Autodesk Fusion 360 part; units mm, degrees
(part 2 of 3)
  spline S66 degree 5 poles (-69.4959, 44.6139) (-69.3858, 44.4624) (-69.2873, 44.0709) (-69.5097, 43.2258) (-70.5375, 41.634) (-72.8973, 39.0758) (-76.0944, 36.2068) (-79.8229, 33.3082) (-83.7318, 30.658) (-87.4483, 28.5038) (-90.6105, 27.0501) (-92.8999, 26.443) (-94.0756, 26.7557) (-94.0097, 27.9705) (-92.7249, 29.9603) (-90.3651, 32.5184) (-87.1679, 35.3874) (-83.4395, 38.286) (-79.5306, 40.9363) (-75.814, 43.0904) (-72.6519, 44.5442) (-70.8204, 45.0298) (-69.9479, 44.9801) (-69.606, 44.7654) (-69.4959, 44.6139) knots 0 0 0 0 0 0 0.05 0.1 0.15 0.2 0.25 0.3 0.35 0.4 0.45 0.5 0.55 0.6 0.65 0.7 0.75 0.8 0.85 0.9 0.95 1 1 1 1 1 1
  line L144 (-69.9146, 45.1902) -> (-69.0772, 44.0376)
  line L145 (-69.9146, 45.1902) -> (-69.0772, 44.0376)
  line L146 (-85.3889, 40.9075) -> (-85.5128, 41.2013)
  spline S67 degree 5 poles (-77.8115, 47.5528) (-77.808, 47.4659) (-77.8969, 47.2932) (-78.3187, 47.042) (-79.4326, 46.738) (-81.582, 46.4414) (-84.2579, 46.2523) (-87.1892, 46.1863) (-90.0921, 46.2497) (-92.6973, 46.4372) (-94.7656, 46.7338) (-96.1037, 47.1154) (-96.5801, 47.5501) (-96.1432, 47.9989) (-94.8404, 48.4163) (-92.7994, 48.7562) (-90.2109, 48.9784) (-87.312, 49.054) (-84.3725, 48.973) (-81.678, 48.7483) (-79.5015, 48.4089) (-78.3613, 48.0774) (-77.9183, 47.815) (-77.8151, 47.6398) (-77.8115, 47.5528) knots 0 0 0 0 0 0 0.05 0.1 0.15 0.2 0.25 0.3 0.35 0.4 0.45 0.5 0.55 0.6 0.65 0.7 0.75 0.8 0.85 0.9 0.95 1 1 1 1 1 1
  line L147 (-77.825, 47.881) -> (-77.7981, 47.2246)
  line L148 (-53.2432, 64.6583) -> (-52.9372, 64.4734)
  line L149 (-105.9017, 18.1636) -> (-105.9017, 76.9421)
  spline S68 degree 5 poles (-85.4509, 54.0512) (-85.4681, 54.0103) (-85.5538, 53.9424) (-85.8347, 53.8848) (-86.4976, 53.9022) (-87.715, 54.0845) (-89.1941, 54.4186) (-90.7877, 54.882) (-92.3423, 55.4366) (-93.7126, 56.0256) (-94.7704, 56.5824) (-95.4139, 57.0408) (-95.5768, 57.3449) (-95.2387, 57.4591) (-94.4366, 57.3785) (-93.2522, 57.1222) (-91.8004, 56.726) (-90.2181, 56.2359) (-88.6538, 55.702) (-87.2569, 55.1719) (-86.1659, 54.6895) (-85.6291, 54.3726) (-85.4501, 54.1882) (-85.4336, 54.0922) (-85.4509, 54.0512) knots 0 0 0 0 0 0 0.05 0.1 0.15 0.2 0.25 0.3 0.35 0.4 0.45 0.5 0.55 0.6 0.65 0.7 0.75 0.8 0.85 0.9 0.95 1 1 1 1 1 1
  line L150 (-85.3814, 54.2159) -> (-85.5203, 53.8865)
  spline S69 degree 5 poles (-60.4508, 47.5528) (-60.4508, 47.7401) (-60.3005, 48.1148) (-59.6238, 48.6678) (-57.8567, 49.3514) (-54.4439, 50.034) (-50.171, 50.4758) (-45.4508, 50.6293) (-40.7307, 50.4758) (-36.4578, 50.034) (-33.045, 49.3514) (-30.8361, 48.4969) (-30.0687, 47.5528) (-30.8361, 46.6088) (-33.045, 45.7542) (-36.4578, 45.0717) (-40.7307, 44.6299) (-45.4508, 44.4764) (-50.171, 44.6299) (-54.4439, 45.0717) (-57.8567, 45.7542) (-59.6238, 46.4379) (-60.3005, 46.9909) (-60.4508, 47.3655) (-60.4508, 47.5528) knots 0 0 0 0 0 0 0.05 0.1 0.15 0.2 0.25 0.3 0.35 0.4 0.45 0.5 0.55 0.6 0.65 0.7 0.75 0.8 0.85 0.9 0.95 1 1 1 1 1 1
  line L151 (-60.4508, 46.8405) -> (-60.4508, 48.2651)
  line L152 (-65.2797, 26.5381) -> (-65.622, 26.5091)
  line L153 (-85.3814, 54.2159) -> (-85.5203, 53.8865)
  spline S70 degree 5 poles (-65.4508, 26.5236) (-65.4952, 26.5198) (-65.5861, 26.4593) (-65.7277, 26.2099) (-65.916, 25.5741) (-66.1189, 24.36) (-66.2582, 22.85) (-66.3099, 21.1912) (-66.2628, 19.5413) (-66.1261, 18.0561) (-65.9235, 16.878) (-65.6864, 16.1243) (-65.4475, 15.8754) (-65.2344, 16.1617) (-65.0631, 16.9495) (-64.9409, 18.1551) (-64.8691, 19.6583) (-64.8463, 21.3145) (-64.8707, 22.9673) (-64.9431, 24.4596) (-65.0647, 25.6463) (-65.2003, 26.2547) (-65.3203, 26.4819) (-65.4065, 26.5273) (-65.4508, 26.5236) knots 0 0 0 0 0 0 0.05 0.1 0.15 0.2 0.25 0.3 0.35 0.4 0.45 0.5 0.55 0.6 0.65 0.7 0.75 0.8 0.85 0.9 0.95 1 1 1 1 1 1
  line L154 (-65.2797, 26.5381) -> (-65.622, 26.5091)
  line L155 (-100.9017, 21.7963) -> (-100.9017, 73.3094)
  line L156 (-77.9412, 64.4537) -> (-77.6818, 64.678)
  line L157 (-77.9468, 30.6568) -> (-77.6763, 30.4228)
  spline S71 degree 5 poles (-77.8115, 30.5398) (-77.7779, 30.5107) (-77.7398, 30.4083) (-77.7719, 30.1233) (-77.9933, 29.4982) (-78.5428, 28.3967) (-79.3177, 27.0933) (-80.2509, 25.7209) (-81.2587, 24.4138) (-82.2423, 23.2926) (-83.0987, 22.4585) (-83.7335, 21.9882) (-84.0731, 21.9272) (-84.0772, 22.2841) (-83.7527, 23.0221) (-83.143, 24.0693) (-82.3175, 25.3276) (-81.3624, 26.681) (-80.3712, 28.0037) (-79.4355, 29.1684) (-78.6395, 30.057) (-78.1723, 30.4696) (-77.9416, 30.5828) (-77.8452, 30.5689) (-77.8115, 30.5398) knots 0 0 0 0 0 0 0.05 0.1 0.15 0.2 0.25 0.3 0.35 0.4 0.45 0.5 0.55 0.6 0.65 0.7 0.75 0.8 0.85 0.9 0.95 1 1 1 1 1 1
  line L158 (-77.9468, 30.6568) -> (-77.6763, 30.4228)
  spline S72 degree 5 poles (-69.4959, 50.4918) (-69.606, 50.3402) (-69.9479, 50.1255) (-70.8204, 50.0759) (-72.6519, 50.5615) (-75.814, 52.0152) (-79.5306, 54.1694) (-83.4395, 56.8197) (-87.1679, 59.7182) (-90.3651, 62.5872) (-92.7249, 65.1454) (-94.0097, 67.1351) (-94.0756, 68.3499) (-92.8999, 68.6626) (-90.6105, 68.0556) (-87.4483, 66.6018) (-83.7318, 64.4477) (-79.8229, 61.7974) (-76.0944, 58.8988) (-72.8973, 56.0298) (-70.5375, 53.4717) (-69.5097, 51.8799) (-69.2873, 51.0348) (-69.3858, 50.6433) (-69.4959, 50.4918) knots 0 0 0 0 0 0 0.05 0.1 0.15 0.2 0.25 0.3 0.35 0.4 0.45 0.5 0.55 0.6 0.65 0.7 0.75 0.8 0.85 0.9 0.95 1 1 1 1 1 1
  line L159 (-69.054, 51.1) -> (-69.9378, 49.8835)
  spline S73 degree 5 poles (-69.2705, 35.7971) (-69.1867, 35.7736) (-69.0499, 35.6357) (-68.9414, 35.1569) (-68.9965, 34.0036) (-69.3786, 31.8677) (-70.0256, 29.2644) (-70.8688, 26.4561) (-71.8261, 23.7149) (-72.8095, 21.2952) (-73.7307, 19.4197) (-74.5071, 18.265) (-75.0678, 17.9463) (-75.3596, 18.5006) (-75.3539, 19.8685) (-75.0465, 21.9147) (-74.4579, 24.4452) (-73.634, 27.2255) (-72.6486, 29.9961) (-71.6023, 32.4893) (-70.607, 34.4544) (-69.9393, 35.4364) (-69.5529, 35.7766) (-69.3543, 35.8206) (-69.2705, 35.7971) knots 0 0 0 0 0 0 0.05 0.1 0.15 0.2 0.25 0.3 0.35 0.4 0.45 0.5 0.55 0.6 0.65 0.7 0.75 0.8 0.85 0.9 0.95 1 1 1 1 1 1
  line L160 (-69.6009, 35.8897) -> (-68.9401, 35.7046)
  line L161 (-69.6009, 35.8897) -> (-68.9401, 35.7046)
  line L162 (-77.825, 47.881) -> (-77.7981, 47.2246)
  line L163 (-40.8441, 29.2615) -> (-40.4508, 29.3893)
  line L164 (-51.9098, 5.8779) -> (-100.9017, 21.7963)
  spline S74 degree 5 poles (-69.2705, 59.3085) (-69.3521, 59.2783) (-69.5439, 59.3095) (-69.9131, 59.6331) (-70.5464, 60.5985) (-71.4927, 62.551) (-72.4994, 65.0375) (-73.468, 67.805) (-74.3048, 70.5854) (-74.9314, 73.121) (-75.2885, 75.1797) (-75.3391, 76.5703) (-75.0729, 77.1577) (-74.511, 76.8808) (-73.7115, 75.7708) (-72.7575, 73.9347) (-71.7463, 71.5415) (-70.7786, 68.8079) (-69.9473, 65.9873) (-69.3284, 63.3552) (-68.9785, 61.1804) (-68.9415, 59.9935) (-69.0542, 59.4911) (-69.1889, 59.3388) (-69.2705, 59.3085) knots 0 0 0 0 0 0 0.05 0.1 0.15 0.2 0.25 0.3 0.35 0.4 0.45 0.5 0.55 0.6 0.65 0.7 0.75 0.8 0.85 0.9 0.95 1 1 1 1 1 1
  line L165 (-68.9863, 59.4139) -> (-69.5547, 59.2031)
  line L166 (-53.2371, 30.451) -> (-52.9432, 30.6286)
  line L167 (-65.4508, 47.5528) -> (-75.4308, 78.2679) construction
  spline S75 degree 5 poles (-53.0902, 30.5398) (-53.0521, 30.5628) (-52.943, 30.5674) (-52.6818, 30.4488) (-52.1557, 30.0451) (-51.278, 29.1821) (-50.2777, 28.0423) (-49.2609, 26.7307) (-48.3292, 25.3683) (-47.5668, 24.0864) (-47.0383, 23.0142) (-46.7871, 22.265) (-46.8341, 21.9233) (-47.1747, 22.0296) (-47.7763, 22.5663) (-48.5839, 23.4698) (-49.5255, 24.6437) (-50.5175, 25.9702) (-51.4692, 27.3217) (-52.2878, 28.5716) (-52.8869, 29.6031) (-53.1349, 30.175) (-53.1713, 30.4294) (-53.1282, 30.5168) (-53.0902, 30.5398) knots 0 0 0 0 0 0 0.05 0.1 0.15 0.2 0.25 0.3 0.35 0.4 0.45 0.5 0.55 0.6 0.65 0.7 0.75 0.8 0.85 0.9 0.95 1 1 1 1 1 1
  line L168 (-53.2371, 30.451) -> (-52.9432, 30.6286)
  spline S76 degree 5 poles (-55.4508, 40.2874) (-55.4026, 40.3599) (-55.2291, 40.4473) (-54.7402, 40.4026) (-53.6604, 39.9937) (-51.7472, 38.9703) (-49.4712, 37.5505) (-47.0609, 35.8808) (-44.7497, 34.1233) (-42.7523, 32.4403) (-41.2533, 30.9846) (-40.3951, 29.8894) (-40.2652, 29.2577) (-40.8825, 29.1514) (-42.1818, 29.5795) (-44.0327, 30.5042) (-46.2575, 31.8459) (-48.6472, 33.4887) (-50.9776, 35.282) (-53.0254, 37.0476) (-54.5868, 38.6014) (-55.3144, 39.5399) (-55.5185, 40.0125) (-55.4991, 40.2149) (-55.4508, 40.2874) knots 0 0 0 0 0 0 0.05 0.1 0.15 0.2 0.25 0.3 0.35 0.4 0.45 0.5 0.55 0.6 0.65 0.7 0.75 0.8 0.85 0.9 0.95 1 1 1 1 1 1
  line L169 (-55.6409, 40.0018) -> (-55.2608, 40.573)
  line L170 (-64.5176, 42.5988) -> (-63.2939, 42.9963)
  spline S77 degree 5 poles (-63.9058, 52.3081) (-64.0839, 52.366) (-64.3937, 52.6248) (-64.7106, 53.4392) (-64.8147, 55.3311) (-64.4092, 58.7878) (-63.509, 62.9881) (-62.1964, 67.5246) (-60.5918, 71.9663) (-58.8512, 75.8936) (-57.1475, 78.9284) (-55.6521, 80.7651) (-54.5172, 81.2032) (-53.8565, 80.1817) (-53.7263, 77.8168) (-54.1318, 74.3602) (-55.032, 70.1598) (-56.3447, 65.6233) (-57.9492, 61.1816) (-59.6898, 57.2543) (-61.3935, 54.2195) (-62.5898, 52.7501) (-63.3249, 52.2775) (-63.7276, 52.2502) (-63.9058, 52.3081) knots 0 0 0 0 0 0 0.05 0.1 0.15 0.2 0.25 0.3 0.35 0.4 0.45 0.5 0.55 0.6 0.65 0.7 0.75 0.8 0.85 0.9 0.95 1 1 1 1 1 1
  line L171 (-63.1907, 52.0758) -> (-64.6208, 52.5404)
  line L172 (-45.4146, 53.896) -> (-45.4871, 54.2065)
  line L173 (-65.28, 68.5676) -> (-65.6217, 68.5966)
  line L174 (-69.054, 51.1) -> (-69.9378, 49.8835)
  line L175 (-55.6409, 40.0018) -> (-55.2608, 40.573)
  line L176 (-51.9098, 89.2278) -> (-21.6312, 47.5528)
  spline S78 degree 5 poles (-63.9058, 42.7975) (-63.7276, 42.8554) (-63.3249, 42.8282) (-62.5898, 42.3555) (-61.3935, 40.8861) (-59.6898, 37.8513) (-57.9492, 33.9241) (-56.3447, 29.4824) (-55.032, 24.9458) (-54.1318, 20.7455) (-53.7263, 17.2889) (-53.8565, 14.9239) (-54.5172, 13.9024) (-55.6521, 14.3405) (-57.1475, 16.1773) (-58.8512, 19.2121) (-60.5918, 23.1393) (-62.1964, 27.581) (-63.509, 32.1176) (-64.4092, 36.3179) (-64.8147, 39.7745) (-64.7106, 41.6665) (-64.3937, 42.4809) (-64.0839, 42.7397) (-63.9058, 42.7975) knots 0 0 0 0 0 0 0.05 0.1 0.15 0.2 0.25 0.3 0.35 0.4 0.45 0.5 0.55 0.6 0.65 0.7 0.75 0.8 0.85 0.9 0.95 1 1 1 1 1 1
  line L177 (-64.5176, 42.5988) -> (-63.2939, 42.9963)
  spline S79 degree 5 poles (-45.4508, 41.0544) (-45.461, 41.0111) (-45.4316, 40.9059) (-45.2381, 40.6942) (-44.6916, 40.3186) (-43.5996, 39.7505) (-42.2065, 39.1514) (-40.6449, 38.5896) (-39.0612, 38.1246) (-37.6065, 37.7956) (-36.4234, 37.6243) (-35.6333, 37.6169) (-35.3228, 37.7672) (-35.5292, 38.0583) (-36.2255, 38.4646) (-37.3344, 38.9534) (-38.7418, 39.4862) (-40.3099, 40.0197) (-41.8893, 40.5073) (-43.331, 40.8995) (-44.4972, 41.1505) (-45.1177, 41.2097) (-45.3709, 41.1657) (-45.4407, 41.0977) (-45.4508, 41.0544) knots 0 0 0 0 0 0 0.05 0.1 0.15 0.2 0.25 0.3 0.35 0.4 0.45 0.5 0.55 0.6 0.65 0.7 0.75 0.8 0.85 0.9 0.95 1 1 1 1 1 1
  line L178 (-45.4118, 41.2217) -> (-45.4899, 40.8872)
  line L179 (37.2139, 59.8404) -> (37.5074, 60.0178)
  line L180 (20.8643, 65.2749) -> (21.4964, 65.0978)
  line L181 (25.8301, 71.9545) -> (27.2601, 72.4191)
  line L182 (-10.4508, 51.1855) -> (-10.4508, 102.6986)
  spline S80 degree 5 poles (21.1803, 65.1864) (21.2642, 65.1629) (21.4009, 65.0249) (21.5095, 64.5461) (21.4543, 63.3929) (21.0722, 61.257) (20.4252, 58.6537) (19.5821, 55.8454) (18.6248, 53.1042) (17.6414, 50.6845) (16.7202, 48.809) (15.9438, 47.6543) (15.3831, 47.3356) (15.0913, 47.8898) (15.0969, 49.2578) (15.4043, 51.3039) (15.9929, 53.8344) (16.8168, 56.6148) (17.8023, 59.3853) (18.8486, 61.8785) (19.8439, 63.8436) (20.5115, 64.8256) (20.898, 65.1658) (21.0965, 65.2099) (21.1803, 65.1864) knots 0 0 0 0 0 0 0.05 0.1 0.15 0.2 0.25 0.3 0.35 0.4 0.45 0.5 0.55 0.6 0.65 0.7 0.75 0.8 0.85 0.9 0.95 1 1 1 1 1 1
  line L183 (20.8643, 65.2749) -> (21.4964, 65.0978)
  spline S81 degree 5 poles (5, 70.4437) (4.9827, 70.4847) (4.8971, 70.5525) (4.6162, 70.6101) (3.9532, 70.5927) (2.7358, 70.4104) (1.2567, 70.0763) (-0.3369, 69.6129) (-1.8915, 69.0583) (-3.2617, 68.4693) (-4.3196, 67.9125) (-4.9631, 67.4541) (-5.126, 67.15) (-4.7879, 67.0358) (-3.9857, 67.1164) (-2.8013, 67.3727) (-1.3495, 67.7689) (0.2327, 68.259) (1.7971, 68.7929) (3.1939, 69.323) (4.285, 69.8054) (4.8217, 70.1223) (5.0007, 70.3067) (5.0173, 70.4027) (5, 70.4437) knots 0 0 0 0 0 0 0.05 0.1 0.15 0.2 0.25 0.3 0.35 0.4 0.45 0.5 0.55 0.6 0.65 0.7 0.75 0.8 0.85 0.9 0.95 1 1 1 1 1 1
  line L184 (5.0667, 70.2855) -> (4.9333, 70.6019)
  line L185 (25.1781, 55.928) -> (24.8219, 55.8977)
  line L186 (20.5362, 74.5794) -> (21.3736, 73.4269)
  line L187 (21.333, 80.4015) -> (20.5768, 79.3606)
  line L188 (-5.6587, 77.2766) -> (-5.9017, 76.9421)
  line L189 (5.0667, 70.2855) -> (4.9333, 70.6019)
  line L190 (12.5187, 60.0334) -> (12.7599, 59.8248)
  spline S82 degree 5 poles (12.6393, 76.9421) (12.6429, 76.8551) (12.5539, 76.6824) (12.1321, 76.4312) (11.0182, 76.1273) (8.8688, 75.8307) (6.193, 75.6415) (3.2616, 75.5756) (0.3587, 75.639) (-2.2464, 75.8265) (-4.3148, 76.1231) (-5.6529, 76.5047) (-6.1293, 76.9394) (-5.6923, 77.3882) (-4.3895, 77.8056) (-2.3486, 78.1455) (0.24, 78.3677) (3.1388, 78.4433) (6.0783, 78.3622) (8.7728, 78.1375) (10.9493, 77.7982) (12.0895, 77.4667) (12.5325, 77.2043) (12.6357, 77.0291) (12.6393, 76.9421) knots 0 0 0 0 0 0 0.05 0.1 0.15 0.2 0.25 0.3 0.35 0.4 0.45 0.5 0.55 0.6 0.65 0.7 0.75 0.8 0.85 0.9 0.95 1 1 1 1 1 1
  line L191 (12.6252, 77.2849) -> (12.6534, 76.5993)
  spline S83 degree 5 poles (26.5451, 72.1868) (26.7232, 72.2447) (27.126, 72.2174) (27.861, 71.7448) (29.0573, 70.2754) (30.7611, 67.2406) (32.5016, 63.3133) (34.1062, 58.8716) (35.4188, 54.3351) (36.3191, 50.1348) (36.7245, 46.6781) (36.5944, 44.3132) (35.9337, 43.2917) (34.7987, 43.7298) (33.3034, 45.5665) (31.5996, 48.6013) (29.8591, 52.5286) (28.2545, 56.9703) (26.9418, 61.5068) (26.0416, 65.7072) (25.6361, 69.1638) (25.7403, 71.0557) (26.0571, 71.8701) (26.3669, 72.1289) (26.5451, 72.1868) knots 0 0 0 0 0 0 0.05 0.1 0.15 0.2 0.25 0.3 0.35 0.4 0.45 0.5 0.55 0.6 0.65 0.7 0.75 0.8 0.85 0.9 0.95 1 1 1 1 1 1
  line L192 (25.8301, 71.9545) -> (27.2601, 72.4191)
  line L193 (38.541, 35.2671) -> (-10.4508, 51.1855)
  line L194 (25, 76.9421) -> (51.1278, 57.9592) construction
  spline S84 degree 5 poles (12.6393, 59.9291) (12.6729, 59.9) (12.711, 59.7976) (12.679, 59.5126) (12.4575, 58.8875) (11.908, 57.786) (11.1332, 56.4825) (10.2, 55.1101) (9.1921, 53.803) (8.2086, 52.6818) (7.3521, 51.8478) (6.7173, 51.3775) (6.3777, 51.3165) (6.3736, 51.6733) (6.6981, 52.4113) (7.3079, 53.4586) (8.1333, 54.7169) (9.0884, 56.0702) (10.0796, 57.393) (11.0154, 58.5577) (11.8113, 59.4463) (12.2786, 59.8588) (12.5092, 59.9721) (12.6057, 59.9582) (12.6393, 59.9291) knots 0 0 0 0 0 0 0.05 0.1 0.15 0.2 0.25 0.3 0.35 0.4 0.45 0.5 0.55 0.6 0.65 0.7 0.75 0.8 0.85 0.9 0.95 1 1 1 1 1 1
  line L195 (12.5187, 60.0334) -> (12.7599, 59.8248)
  spline S85 degree 5 poles (25, 55.9128) (24.9557, 55.9091) (24.8647, 55.8486) (24.7231, 55.5992) (24.5348, 54.9633) (24.332, 53.7492) (24.1927, 52.2393) (24.141, 50.5804) (24.188, 48.9306) (24.3247, 47.4454) (24.5274, 46.2672) (24.7645, 45.5136) (25.0034, 45.2647) (25.2164, 45.5509) (25.3877, 46.3387) (25.51, 47.5444) (25.5818, 49.0475) (25.6046, 50.7038) (25.5802, 52.3565) (25.5077, 53.8488) (25.3861, 55.0356) (25.2506, 55.644) (25.1305, 55.8712) (25.0443, 55.9166) (25, 55.9128) knots 0 0 0 0 0 0 0.05 0.1 0.15 0.2 0.25 0.3 0.35 0.4 0.45 0.5 0.55 0.6 0.65 0.7 0.75 0.8 0.85 0.9 0.95 1 1 1 1 1 1
  line L196 (25.1781, 55.928) -> (24.8219, 55.8977)
  spline S86 degree 5 poles (35, 69.6767) (35.0482, 69.7491) (35.2217, 69.8366) (35.7106, 69.7918) (36.7904, 69.383) (38.7037, 68.3596) (40.9796, 66.9398) (43.3899, 65.2701) (45.7012, 63.5126) (47.6985, 61.8296) (49.1976, 60.3739) (50.0558, 59.2787) (50.1857, 58.6469) (49.5684, 58.5407) (48.2691, 58.9688) (46.4181, 59.8934) (44.1933, 61.2352) (41.8037, 62.8779) (39.4732, 64.6713) (37.4254, 66.4368) (35.864, 67.9907) (35.1364, 68.9291) (34.9323, 69.4018) (34.9518, 69.6042) (35, 69.6767) knots 0 0 0 0 0 0 0.05 0.1 0.15 0.2 0.25 0.3 0.35 0.4 0.45 0.5 0.55 0.6 0.65 0.7 0.75 0.8 0.85 0.9 0.95 1 1 1 1 1 1
  line L197 (34.8321, 69.4244) -> (35.1679, 69.929)
  spline S87 degree 5 poles (37.3607, 59.9291) (37.3987, 59.9521) (37.5079, 59.9566) (37.769, 59.8381) (38.2951, 59.4343) (39.1729, 58.5713) (40.1731, 57.4316) (41.19, 56.12) (42.1217, 54.7575) (42.884, 53.4756) (43.4126, 52.4034) (43.6637, 51.6543) (43.6168, 51.3125) (43.2761, 51.4189) (42.6745, 51.9556) (41.867, 52.8591) (40.9253, 54.033) (39.9334, 55.3595) (38.9816, 56.7109) (38.1631, 57.9608) (37.564, 58.9924) (37.316, 59.5643) (37.2796, 59.8186) (37.3226, 59.9061) (37.3607, 59.9291) knots 0 0 0 0 0 0 0.05 0.1 0.15 0.2 0.25 0.3 0.35 0.4 0.45 0.5 0.55 0.6 0.65 0.7 0.75 0.8 0.85 0.9 0.95 1 1 1 1 1 1
  line L198 (37.2139, 59.8404) -> (37.5074, 60.0178)
  spline S88 degree 5 poles (45, 83.4405) (44.9899, 83.4838) (45.0193, 83.589) (45.2127, 83.8007) (45.7593, 84.1763) (46.8513, 84.7444) (48.2443, 85.3435) (49.806, 85.9053) (51.3896, 86.3704) (52.8444, 86.6993) (54.0275, 86.8706) (54.8175, 86.878) (55.1281, 86.7277) (54.9216, 86.4366) (54.2253, 86.0303) (53.1165, 85.5415) (51.7091, 85.0087) (50.1409, 84.4752) (48.5615, 83.9876) (47.1199, 83.5954) (45.9537, 83.3444) (45.3331, 83.2853) (45.08, 83.3292) (45.0101, 83.3972) (45, 83.4405) knots 0 0 0 0 0 0 0.05 0.1 0.15 0.2 0.25 0.3 0.35 0.4 0.45 0.5 0.55 0.6 0.65 0.7 0.75 0.8 0.85 0.9 0.95 1 1 1 1 1 1
  line L199 (45.0407, 83.2664) -> (44.9593, 83.6146)
  line L200 (21.5021, 88.8171) -> (20.8586, 88.5785)
  line L201 (45.0407, 83.2664) -> (44.9593, 83.6146)
  line L202 (25.1782, 97.9562) -> (24.8218, 97.9865)
  line L203 (37.2242, 94.0376) -> (37.4971, 93.8726)
  spline S89 degree 5 poles (26.5451, 81.6974) (26.3669, 81.7553) (26.0571, 82.014) (25.7403, 82.8285) (25.6361, 84.7204) (26.0416, 88.177) (26.9418, 92.3773) (28.2545, 96.9139) (29.8591, 101.3556) (31.5996, 105.2829) (33.3034, 108.3177) (34.7987, 110.1544) (35.9337, 110.5925) (36.5944, 109.571) (36.7245, 107.2061) (36.3191, 103.7494) (35.4188, 99.5491) (34.1062, 95.0126) (32.5016, 90.5709) (30.7611, 86.6436) (29.0573, 83.6088) (27.861, 82.1394) (27.126, 81.6667) (26.7232, 81.6395) (26.5451, 81.6974) knots 0 0 0 0 0 0 0.05 0.1 0.15 0.2 0.25 0.3 0.35 0.4 0.45 0.5 0.55 0.6 0.65 0.7 0.75 0.8 0.85 0.9 0.95 1 1 1 1 1 1
  line L204 (27.2225, 81.4773) -> (25.8676, 81.9175)
  spline S90 degree 5 poles (21.1803, 88.6978) (21.0987, 88.6675) (20.907, 88.6987) (20.5377, 89.0223) (19.9045, 89.9877) (18.9582, 91.9403) (17.9514, 94.4267) (16.9829, 97.1942) (16.1461, 99.9746) (15.5194, 102.5102) (15.1623, 104.569) (15.1117, 105.9595) (15.378, 106.5469) (15.9398, 106.2701) (16.7393, 105.16) (17.6933, 103.324) (18.7045, 100.9308) (19.6722, 98.1972) (20.5035, 95.3765) (21.1225, 92.7445) (21.4723, 90.5696) (21.5094, 89.3828) (21.3967, 88.8804) (21.262, 88.7281) (21.1803, 88.6978) knots 0 0 0 0 0 0 0.05 0.1 0.15 0.2 0.25 0.3 0.35 0.4 0.45 0.5 0.55 0.6 0.65 0.7 0.75 0.8 0.85 0.9 0.95 1 1 1 1 1 1
  line L205 (21.5021, 88.8171) -> (20.8586, 88.5785)
  line L206 (68.8197, 76.9421) -> (38.541, 35.2671)
  line L207 (45.039, 70.6107) -> (44.961, 70.2767)
  line L208 (40.4508, 124.4949) -> (75, 76.9421)
  spline S91 degree 5 poles (35, 84.2075) (34.946, 84.2758) (34.9164, 84.4678) (35.1101, 84.9189) (35.8326, 85.8195) (37.3971, 87.3229) (39.4507, 89.0487) (41.7835, 90.8251) (44.1692, 92.4801) (46.3871, 93.8597) (48.2347, 94.8355) (49.5416, 95.3133) (50.1825, 95.2416) (50.0928, 94.6217) (49.2842, 93.5183) (47.8328, 92.0436) (45.8692, 90.3424) (43.5684, 88.5773) (41.1427, 86.9151) (38.8307, 85.5131) (36.8705, 84.5083) (35.7531, 84.1063) (35.2405, 84.0582) (35.054, 84.1393) (35, 84.2075) knots 0 0 0 0 0 0 0.05 0.1 0.15 0.2 0.25 0.3 0.35 0.4 0.45 0.5 0.55 0.6 0.65 0.7 0.75 0.8 0.85 0.9 0.95 1 1 1 1 1 1
  line L209 (35.2038, 83.9499) -> (34.7962, 84.4651)
  spline S92 degree 5 poles (30, 76.9421) (30, 77.1294) (30.1504, 77.504) (30.827, 78.057) (32.5942, 78.7407) (36.0069, 79.4233) (40.2799, 79.865) (45, 80.0185) (49.7201, 79.865) (53.9931, 79.4233) (57.4058, 78.7407) (59.6148, 77.8861) (60.3821, 76.9421) (59.6148, 75.9981) (57.4058, 75.1435) (53.9931, 74.4609) (49.7201, 74.0191) (45, 73.8657) (40.2799, 74.0191) (36.0069, 74.4609) (32.5942, 75.1435) (30.827, 75.8271) (30.1504, 76.3801) (30, 76.7548) (30, 76.9421) knots 0 0 0 0 0 0 0.05 0.1 0.15 0.2 0.25 0.3 0.35 0.4 0.45 0.5 0.55 0.6 0.65 0.7 0.75 0.8 0.85 0.9 0.95 1 1 1 1 1 1
  line L210 (30, 76.1903) -> (30, 77.6939)
  line L211 (35.2038, 83.9499) -> (34.7962, 84.4651)
  spline S93 degree 5 poles (37.3607, 93.9551) (37.3987, 93.9321) (37.5079, 93.9276) (37.769, 94.0461) (38.2951, 94.4499) (39.1729, 95.3129) (40.1731, 96.4526) (41.19, 97.7642) (42.1217, 99.1266) (42.884, 100.4085) (43.4126, 101.4808) (43.6637, 102.2299) (43.6168, 102.5716) (43.2761, 102.4653) (42.6745, 101.9286) (41.867, 101.0251) (40.9253, 99.8512) (39.9334, 98.5247) (38.9816, 97.1732) (38.1631, 95.9234) (37.564, 94.8918) (37.316, 94.3199) (37.2796, 94.0655) (37.3226, 93.9781) (37.3607, 93.9551) knots 0 0 0 0 0 0 0.05 0.1 0.15 0.2 0.25 0.3 0.35 0.4 0.45 0.5 0.55 0.6 0.65 0.7 0.75 0.8 0.85 0.9 0.95 1 1 1 1 1 1
  line L212 (37.2242, 94.0376) -> (37.4971, 93.8726)
  line L213 (27.2225, 81.4773) -> (25.8676, 81.9175)
  spline S94 degree 5 poles (25, 97.9713) (24.9557, 97.9751) (24.8647, 98.0356) (24.7231, 98.285) (24.5348, 98.9209) (24.332, 100.135) (24.1927, 101.6449) (24.141, 103.3037) (24.188, 104.9536) (24.3247, 106.4388) (24.5274, 107.6169) (24.7645, 108.3706) (25.0034, 108.6195) (25.2164, 108.3332) (25.3877, 107.5454) (25.51, 106.3398) (25.5818, 104.8366) (25.6046, 103.1804) (25.5802, 101.5276) (25.5077, 100.0353) (25.3861, 98.8486) (25.2506, 98.2402) (25.1305, 98.013) (25.0443, 97.9676) (25, 97.9713) knots 0 0 0 0 0 0 0.05 0.1 0.15 0.2 0.25 0.3 0.35 0.4 0.45 0.5 0.55 0.6 0.65 0.7 0.75 0.8 0.85 0.9 0.95 1 1 1 1 1 1
  line L214 (25.1782, 97.9562) -> (24.8218, 97.9865)
  line L215 (12.5094, 93.8428) -> (12.7692, 94.0674)
  line L216 (38.541, 118.6171) -> (68.8197, 76.9421)
  spline S95 degree 5 poles (12.6393, 93.9551) (12.6729, 93.9842) (12.711, 94.0866) (12.679, 94.3716) (12.4575, 94.9967) (11.908, 96.0982) (11.1332, 97.4016) (10.2, 98.774) (9.1921, 100.0812) (8.2086, 101.2023) (7.3521, 102.0364) (6.7173, 102.5067) (6.3777, 102.5677) (6.3736, 102.2108) (6.6981, 101.4728) (7.3079, 100.4256) (8.1333, 99.1673) (9.0884, 97.814) (10.0796, 96.4912) (11.0154, 95.3265) (11.8113, 94.4379) (12.2786, 94.0253) (12.5092, 93.9121) (12.6057, 93.926) (12.6393, 93.9551) knots 0 0 0 0 0 0 0.05 0.1 0.15 0.2 0.25 0.3 0.35 0.4 0.45 0.5 0.55 0.6 0.65 0.7 0.75 0.8 0.85 0.9 0.95 1 1 1 1 1 1
  line L217 (12.5094, 93.8428) -> (12.7692, 94.0674)
  spline S96 degree 5 poles (45, 70.4437) (44.9899, 70.4004) (45.0193, 70.2952) (45.2127, 70.0835) (45.7593, 69.7079) (46.8513, 69.1398) (48.2443, 68.5407) (49.806, 67.9789) (51.3896, 67.5138) (52.8444, 67.1849) (54.0275, 67.0135) (54.8175, 67.0062) (55.1281, 67.1564) (54.9216, 67.4475) (54.2253, 67.8539) (53.1165, 68.3427) (51.7091, 68.8755) (50.1409, 69.409) (48.5615, 69.8965) (47.1199, 70.2888) (45.9537, 70.5398) (45.3331, 70.5989) (45.08, 70.5549) (45.0101, 70.487) (45, 70.4437) knots 0 0 0 0 0 0 0.05 0.1 0.15 0.2 0.25 0.3 0.35 0.4 0.45 0.5 0.55 0.6 0.65 0.7 0.75 0.8 0.85 0.9 0.95 1 1 1 1 1 1
  line L218 (45.039, 70.6107) -> (44.961, 70.2767)
  line L219 (5.0667, 83.5987) -> (4.9333, 83.2822)
  spline S97 degree 5 poles (20.9549, 79.881) (20.8448, 79.7295) (20.503, 79.5148) (19.6305, 79.4651) (17.799, 79.9507) (14.6368, 81.4045) (10.9203, 83.5586) (7.0114, 86.2089) (3.2829, 89.1075) (0.0857, 91.9765) (-2.2741, 94.5346) (-3.5588, 96.5244) (-3.6247, 97.7392) (-2.449, 98.0519) (-0.1597, 97.4449) (3.0025, 95.9911) (6.719, 93.8369) (10.6279, 91.1867) (14.3564, 88.2881) (17.5536, 85.4191) (19.9134, 82.8609) (20.9412, 81.2691) (21.1636, 80.424) (21.065, 80.0326) (20.9549, 79.881) knots 0 0 0 0 0 0 0.05 0.1 0.15 0.2 0.25 0.3 0.35 0.4 0.45 0.5 0.55 0.6 0.65 0.7 0.75 0.8 0.85 0.9 0.95 1 1 1 1 1 1
  line L220 (21.333, 80.4015) -> (20.5768, 79.3606)
  line L221 (30, 76.1903) -> (30, 77.6939)
  spline S98 degree 5 poles (5, 83.4405) (4.9827, 83.3995) (4.8971, 83.3317) (4.6162, 83.2741) (3.9532, 83.2915) (2.7358, 83.4737) (1.2567, 83.8079) (-0.3369, 84.2713) (-1.8915, 84.8259) (-3.2617, 85.4149) (-4.3196, 85.9716) (-4.9631, 86.4301) (-5.126, 86.7342) (-4.7879, 86.8483) (-3.9857, 86.7678) (-2.8013, 86.5115) (-1.3495, 86.1153) (0.2327, 85.6252) (1.7971, 85.0912) (3.1939, 84.5612) (4.285, 84.0788) (4.8217, 83.7619) (5.0007, 83.5775) (5.0173, 83.4815) (5, 83.4405) knots 0 0 0 0 0 0 0.05 0.1 0.15 0.2 0.25 0.3 0.35 0.4 0.45 0.5 0.55 0.6 0.65 0.7 0.75 0.8 0.85 0.9 0.95 1 1 1 1 1 1
  line L222 (5.0667, 83.5987) -> (4.9333, 83.2822)
  line L223 (-10.4508, 102.6986) -> (38.541, 118.6171)
  line L224 (-15.4508, 47.5528) -> (-15.4508, 106.3314)
  line L225 (-15.4508, 106.3314) -> (40.4508, 124.4949)
  line L226 (-5, 86.6897) -> (-5.715, 86.922)
  line L227 (8.2319, 87.8888) -> (7.0563, 86.2707)
  line L228 (12.6252, 77.2849) -> (12.6534, 76.5993)
  line L229 (-4.9757, 86.7231) -> (-5, 86.6897)
  spline S99 degree 5 poles (20.9549, 74.0032) (21.065, 73.8516) (21.1636, 73.4602) (20.9412, 72.615) (19.9134, 71.0232) (17.5536, 68.4651) (14.3564, 65.5961) (10.6279, 62.6975) (6.719, 60.0472) (3.0025, 57.8931) (-0.1597, 56.4393) (-2.449, 55.8323) (-3.6247, 56.145) (-3.5588, 57.3598) (-2.2741, 59.3495) (0.0857, 61.9077) (3.2829, 64.7767) (7.0114, 67.6753) (10.9203, 70.3255) (14.6368, 72.4797) (17.799, 73.9335) (19.6305, 74.4191) (20.503, 74.3694) (20.8448, 74.1547) (20.9549, 74.0032) knots 0 0 0 0 0 0 0.05 0.1 0.15 0.2 0.25 0.3 0.35 0.4 0.45 0.5 0.55 0.6 0.65 0.7 0.75 0.8 0.85 0.9 0.95 1 1 1 1 1 1
  line L230 (20.5362, 74.5794) -> (21.3736, 73.4269)
  line L231 (75, 76.9421) -> (40.4508, 29.3893)
  line L232 (34.8321, 69.4244) -> (35.1679, 69.929)
  spline S100 degree 5 poles (76.8566, 2.9389) (76.7465, 2.7874) (76.4047, 2.5727) (75.5322, 2.523) (73.7007, 3.0086) (70.5385, 4.4624) (66.822, 6.6166) (62.9131, 9.2668) (59.1846, 12.1654) (55.9874, 15.0344) (53.6276, 17.5926) (52.3429, 19.5823) (52.277, 20.7971) (53.4527, 21.1098) (55.742, 20.5028) (58.9042, 19.049) (62.6207, 16.8949) (66.5296, 14.2446) (70.2581, 11.346) (73.4553, 8.477) (75.8151, 5.9189) (76.8429, 4.327) (77.0653, 3.4819) (76.9667, 3.0905) (76.8566, 2.9389) knots 0 0 0 0 0 0 0.05 0.1 0.15 0.2 0.25 0.3 0.35 0.4 0.45 0.5 0.55 0.6 0.65 0.7 0.75 0.8 0.85 0.9 0.95 1 1 1 1 1 1
  line L233 (77.2985, 3.5472) -> (76.4147, 2.3307)
  spline S101 degree 5 poles (93.2624, 17.013) (93.3004, 16.99) (93.4096, 16.9855) (93.6707, 17.104) (94.1968, 17.5078) (95.0746, 18.3708) (96.0748, 19.5105) (97.0917, 20.8221) (98.0234, 22.1845) (98.7857, 23.4664) (99.3143, 24.5387) (99.5654, 25.2878) (99.5185, 25.6296) (99.1778, 25.5232) (98.5762, 24.9865) (97.7687, 24.083) (96.827, 22.9091) (95.8351, 21.5826) (94.8833, 20.2311) (94.0648, 18.9813) (93.4657, 17.9497) (93.2177, 17.3778) (93.1813, 17.1234) (93.2243, 17.036) (93.2624, 17.013) knots 0 0 0 0 0 0 0.05 0.1 0.15 0.2 0.25 0.3 0.35 0.4 0.45 0.5 0.55 0.6 0.65 0.7 0.75 0.8 0.85 0.9 0.95 1 1 1 1 1 1
  line L234 (93.1154, 17.1018) -> (93.4093, 16.9242)
  spline S102 degree 5 poles (77.082, 11.7557) (77.0004, 11.7254) (76.8087, 11.7567) (76.4394, 12.0802) (75.8062, 13.0457) (74.8599, 14.9982) (73.8531, 17.4846) (72.8846, 20.2521) (72.0478, 23.0326) (71.4211, 25.5681) (71.064, 27.6269) (71.0134, 29.0174) (71.2797, 29.6049) (71.8415, 29.328) (72.641, 28.2179) (73.595, 26.3819) (74.6062, 23.9887) (75.5739, 21.2551) (76.4052, 18.4344) (77.0242, 15.8024) (77.374, 13.6276) (77.4111, 12.4407) (77.2984, 11.9383) (77.1637, 11.786) (77.082, 11.7557) knots 0 0 0 0 0 0 0.05 0.1 0.15 0.2 0.25 0.3 0.35 0.4 0.45 0.5 0.55 0.6 0.65 0.7 0.75 0.8 0.85 0.9 0.95 1 1 1 1 1 1
  line L235 (77.3898, 11.8699) -> (76.7743, 11.6415)
  line L236 (68.4058, 16.8961) -> (68.6762, 17.1299)
  line L237 (83.1242, 4.5352) -> (81.7693, 4.9754)
  spline S103 degree 5 poles (100.9017, 6.4984) (100.8916, 6.5417) (100.921, 6.6469) (101.1144, 6.8586) (101.661, 7.2342) (102.753, 7.8023) (104.146, 8.4014) (105.7077, 8.9632) (107.2913, 9.4283) (108.7461, 9.7572) (109.9292, 9.9285) (110.7192, 9.9359) (111.0298, 9.7856) (110.8233, 9.4946) (110.127, 9.0882) (109.0182, 8.5994) (107.6108, 8.0666) (106.0426, 7.5331) (104.4632, 7.0456) (103.0216, 6.6533) (101.8554, 6.4023) (101.2348, 6.3432) (100.9817, 6.3871) (100.9118, 6.4551) (100.9017, 6.4984) knots 0 0 0 0 0 0 0.05 0.1 0.15 0.2 0.25 0.3 0.35 0.4 0.45 0.5 0.55 0.6 0.65 0.7 0.75 0.8 0.85 0.9 0.95 1 1 1 1 1 1
  line L238 (100.9408, 6.3312) -> (100.8626, 6.6656)
  line L239 (100.9017, 1) -> (100.9017, 3)
  line L240 (105.9017, 17.7501) -> (105.9017, 18.1636)
  line L241 (77.3898, 11.8699) -> (76.7743, 11.6415)
  spline S104 degree 5 poles (80.9017, 21.0292) (80.8574, 21.033) (80.7664, 21.0935) (80.6248, 21.3429) (80.4365, 21.9788) (80.2337, 23.1929) (80.0944, 24.7028) (80.0427, 26.3617) (80.0897, 28.0115) (80.2264, 29.4967) (80.4291, 30.6748) (80.6662, 31.4285) (80.9051, 31.6774) (81.1181, 31.3911) (81.2894, 30.6034) (81.4117, 29.3977) (81.4835, 27.8946) (81.5063, 26.2383) (81.4819, 24.5855) (81.4094, 23.0932) (81.2878, 21.9065) (81.1523, 21.2981) (81.0322, 21.0709) (80.946, 21.0255) (80.9017, 21.0292) knots 0 0 0 0 0 0 0.05 0.1 0.15 0.2 0.25 0.3 0.35 0.4 0.45 0.5 0.55 0.6 0.65 0.7 0.75 0.8 0.85 0.9 0.95 1 1 1 1 1 1
  line L242 (81.0606, 21.0158) -> (80.7428, 21.0427)
  line L243 (110.9017, 9.7063) -> (110.9017, 9.7476)
  line L244 (68.5286, 0.3028) -> (68.5535, -0.3028)
  spline S105 degree 5 poles (68.541, 0) (68.5446, -0.087) (68.4556, -0.2597) (68.0338, -0.5109) (66.9199, -0.8148) (64.7705, -1.1114) (62.0947, -1.3006) (59.1633, -1.3665) (56.2604, -1.3031) (53.6553, -1.1156) (51.5869, -0.819) (50.2488, -0.4374) (49.7724, -0.0027) (50.2094, 0.4461) (51.5122, 0.8635) (53.5531, 1.2034) (56.1417, 1.4256) (59.0405, 1.5012) (61.98, 1.4201) (64.6745, 1.1955) (66.851, 0.8561) (67.9912, 0.5246) (68.4342, 0.2622) (68.5374, 0.087) (68.541, 0) knots 0 0 0 0 0 0 0.05 0.1 0.15 0.2 0.25 0.3 0.35 0.4 0.45 0.5 0.55 0.6 0.65 0.7 0.75 0.8 0.85 0.9 0.95 1 1 1 1 1 1
  line L245 (68.5286, 0.3028) -> (68.5535, -0.3028)
  line L246 (81.0606, 21.0158) -> (80.7428, 21.0427)
  line L247 (91.1146, 6.9964) -> (90.6888, 7.5345)
  line L248 (124.7214, 0) -> (94.4427, -41.675)
  spline S106 degree 5 poles (60.9017, 6.4984) (60.8844, 6.4574) (60.7988, 6.3896) (60.5179, 6.332) (59.8549, 6.3494) (58.6375, 6.5317) (57.1584, 6.8658) (55.5648, 7.3292) (54.0102, 7.8838) (52.64, 8.4728) (51.5821, 9.0296) (50.9386, 9.488) (50.7757, 9.7921) (51.1138, 9.9062) (51.916, 9.8257) (53.1004, 9.5694) (54.5522, 9.1732) (56.1344, 8.6831) (57.6988, 8.1491) (59.0956, 7.6191) (60.1867, 7.1367) (60.7234, 6.8198) (60.9024, 6.6354) (60.919, 6.5394) (60.9017, 6.4984) knots 0 0 0 0 0 0 0.05 0.1 0.15 0.2 0.25 0.3 0.35 0.4 0.45 0.5 0.55 0.6 0.65 0.7 0.75 0.8 0.85 0.9 0.95 1 1 1 1 1 1
  line L249 (60.9683, 6.6564) -> (60.8351, 6.3404)
  spline S107 degree 5 poles (68.541, 17.013) (68.5746, 17.0421) (68.6127, 17.1445) (68.5807, 17.4295) (68.3592, 18.0546) (67.8097, 19.1561) (67.0349, 20.4596) (66.1017, 21.8319) (65.0938, 23.1391) (64.1103, 24.2602) (63.2538, 25.0943) (62.619, 25.5646) (62.2794, 25.6256) (62.2753, 25.2688) (62.5998, 24.5307) (63.2096, 23.4835) (64.035, 22.2252) (64.9901, 20.8719) (65.9813, 19.5491) (66.9171, 18.3844) (67.713, 17.4958) (68.1803, 17.0832) (68.4109, 16.97) (68.5074, 16.9839) (68.541, 17.013) knots 0 0 0 0 0 0 0.05 0.1 0.15 0.2 0.25 0.3 0.35 0.4 0.45 0.5 0.55 0.6 0.65 0.7 0.75 0.8 0.85 0.9 0.95 1 1 1 1 1 1
  line L250 (68.4058, 16.8961) -> (68.6762, 17.1299)
  line L251 (130.9017, 0) -> (96.3525, -47.5528)
  line L252 (96.3525, 47.5528) -> (130.9017, 0)
  line L253 (40.4508, 29.3893) -> (96.3525, 47.5528)
  line L254 (94.4427, 41.675) -> (124.7214, 0)
  spline S108 degree 5 poles (82.4468, 4.7553) (82.2686, 4.8132) (81.9588, 5.0719) (81.642, 5.8864) (81.5378, 7.7783) (81.9433, 11.2349) (82.8435, 15.4352) (84.1562, 19.9718) (85.7608, 24.4135) (87.5013, 28.3408) (89.2051, 31.3756) (90.7004, 33.2123) (91.8354, 33.6504) (92.4961, 32.6289) (92.6262, 30.264) (92.2208, 26.8073) (91.3205, 22.607) (90.0079, 18.0705) (88.4033, 13.6288) (86.6628, 9.7015) (84.959, 6.6667) (83.7627, 5.1973) (83.0277, 4.7246) (82.6249, 4.6974) (82.4468, 4.7553) knots 0 0 0 0 0 0 0.05 0.1 0.15 0.2 0.25 0.3 0.35 0.4 0.45 0.5 0.55 0.6 0.65 0.7 0.75 0.8 0.85 0.9 0.95 1 1 1 1 1 1
  line L255 (83.1242, 4.5352) -> (81.7693, 4.9754)
  line L256 (45.4508, 25.7565) -> (94.4427, 41.675)
  line L257 (110.9017, 9.7476) -> (111.6167, 9.9799)
  line L258 (80.9017, 0) -> (48.606, 0) construction
  spline S109 degree 5 poles (90.9017, 7.2654) (90.8477, 7.3337) (90.8181, 7.5257) (91.0118, 7.9769) (91.7343, 8.8775) (93.2988, 10.3808) (95.3524, 12.1067) (97.6852, 13.883) (100.0709, 15.538) (102.2888, 16.9176) (104.1364, 17.8934) (105.4433, 18.3712) (106.0842, 18.2995) (105.9945, 17.6796) (105.1859, 16.5762) (103.7345, 15.1015) (101.7709, 13.4003) (99.4701, 11.6352) (97.0444, 9.973) (94.7324, 8.571) (92.7722, 7.5662) (91.6548, 7.1642) (91.1422, 7.1161) (90.9557, 7.1972) (90.9017, 7.2654) knots 0 0 0 0 0 0 0.05 0.1 0.15 0.2 0.25 0.3 0.35 0.4 0.45 0.5 0.55 0.6 0.65 0.7 0.75 0.8 0.85 0.9 0.95 1 1 1 1 1 1
  line L259 (91.1146, 6.9964) -> (90.6888, 7.5345)
  line L260 (60.9683, 6.6564) -> (60.8351, 6.3404)
  line L261 (85.9017, -0.6433) -> (85.9017, 0.6433)
  line L262 (93.1154, 17.1018) -> (93.4093, 16.9242)
  line L263 (77.2985, 3.5472) -> (76.4147, 2.3307)
  line L264 (100.9408, 6.3312) -> (100.8626, 6.6656)
  spline S110 degree 5 poles (60.9017, -6.4984) (60.8844, -6.4574) (60.7988, -6.3896) (60.5179, -6.332) (59.8549, -6.3494) (58.6375, -6.5317) (57.1584, -6.8658) (55.5648, -7.3292) (54.0102, -7.8838) (52.64, -8.4728) (51.5821, -9.0296) (50.9386, -9.488) (50.7757, -9.7921) (51.1138, -9.9062) (51.916, -9.8257) (53.1004, -9.5694) (54.5522, -9.1732) (56.1344, -8.6831) (57.6988, -8.1491) (59.0956, -7.6191) (60.1867, -7.1367) (60.7234, -6.8198) (60.9024, -6.6354) (60.919, -6.5394) (60.9017, -6.4984) knots 0 0 0 0 0 0 0.05 0.1 0.15 0.2 0.25 0.3 0.35 0.4 0.45 0.5 0.55 0.6 0.65 0.7 0.75 0.8 0.85 0.9 0.95 1 1 1 1 1 1
  line L265 (60.9683, -6.6564) -> (60.8351, -6.3404)
  line L266 (81.7693, -4.9754) -> (83.1242, -4.5352)
  spline S111 degree 5 poles (85.9017, 0) (85.9017, 0.1873) (86.0521, 0.5619) (86.7287, 1.1149) (88.4959, 1.7986) (91.9086, 2.4812) (96.1816, 2.923) (100.9017, 3.0764) (105.6218, 2.923) (109.8948, 2.4812) (113.3075, 1.7986) (115.5165, 0.944) (116.2838, 0) (115.5165, -0.944) (113.3075, -1.7986) (109.8948, -2.4812) (105.6218, -2.923) (100.9017, -3.0764) (96.1816, -2.923) (91.9086, -2.4812) (88.4959, -1.7986) (86.7287, -1.1149) (86.0521, -0.5619) (85.9017, -0.1873) (85.9017, 0) knots 0 0 0 0 0 0 0.05 0.1 0.15 0.2 0.25 0.3 0.35 0.4 0.45 0.5 0.55 0.6 0.65 0.7 0.75 0.8 0.85 0.9 0.95 1 1 1 1 1 1
  line L267 (85.9017, -0.6433) -> (85.9017, 0.6433)
  spline S112 degree 5 poles (80.9017, -21.0292) (80.8574, -21.033) (80.7664, -21.0935) (80.6248, -21.3429) (80.4365, -21.9788) (80.2337, -23.1929) (80.0944, -24.7028) (80.0427, -26.3617) (80.0897, -28.0115) (80.2264, -29.4967) (80.4291, -30.6748) (80.6662, -31.4285) (80.9051, -31.6774) (81.1181, -31.3911) (81.2894, -30.6034) (81.4117, -29.3977) (81.4835, -27.8946) (81.5063, -26.2383) (81.4819, -24.5855) (81.4094, -23.0932) (81.2878, -21.9065) (81.1523, -21.2981) (81.0322, -21.0709) (80.946, -21.0255) (80.9017, -21.0292) knots 0 0 0 0 0 0 0.05 0.1 0.15 0.2 0.25 0.3 0.35 0.4 0.45 0.5 0.55 0.6 0.65 0.7 0.75 0.8 0.85 0.9 0.95 1 1 1 1 1 1
  line L268 (81.0606, -21.0158) -> (80.7428, -21.0427)
  spline S113 degree 5 poles (68.541, -17.013) (68.5746, -17.0421) (68.6127, -17.1445) (68.5807, -17.4295) (68.3592, -18.0546) (67.8097, -19.1561) (67.0349, -20.4596) (66.1017, -21.8319) (65.0938, -23.1391) (64.1103, -24.2602) (63.2538, -25.0943) (62.619, -25.5646) (62.2794, -25.6256) (62.2753, -25.2688) (62.5998, -24.5307) (63.2096, -23.4835) (64.035, -22.2252) (64.9901, -20.8719) (65.9813, -19.5491) (66.9171, -18.3844) (67.713, -17.4958) (68.1803, -17.0832) (68.4109, -16.97) (68.5074, -16.9839) (68.541, -17.013) knots 0 0 0 0 0 0 0.05 0.1 0.15 0.2 0.25 0.3 0.35 0.4 0.45 0.5 0.55 0.6 0.65 0.7 0.75 0.8 0.85 0.9 0.95 1 1 1 1 1 1
  line L269 (68.4058, -16.8961) -> (68.6762, -17.1299)
  line L270 (60.9683, -6.6564) -> (60.8351, -6.3404)
  line L271 (76.4147, -2.3307) -> (77.2985, -3.5472)
  spline S114 degree 5 poles (90.9017, -7.2654) (90.9499, -7.193) (91.1234, -7.1055) (91.6123, -7.1503) (92.6921, -7.5591) (94.6054, -8.5825) (96.8813, -10.0023) (99.2916, -11.672) (101.6029, -13.4295) (103.6002, -15.1125) (105.0993, -16.5682) (105.9575, -17.6634) (106.0874, -18.2951) (105.4701, -18.4014) (104.1708, -17.9733) (102.3198, -17.0487) (100.095, -15.7069) (97.7054, -14.0642) (95.3749, -12.2708) (93.3271, -10.5052) (91.7657, -8.9514) (91.0381, -8.013) (90.834, -7.5403) (90.8535, -7.3379) (90.9017, -7.2654) knots 0 0 0 0 0 0 0.05 0.1 0.15 0.2 0.25 0.3 0.35 0.4 0.45 0.5 0.55 0.6 0.65 0.7 0.75 0.8 0.85 0.9 0.95 1 1 1 1 1 1
  line L272 (90.7116, -7.5511) -> (91.0918, -6.9798)
  spline S115 degree 5 poles (82.4468, -4.7553) (82.6249, -4.6974) (83.0277, -4.7246) (83.7627, -5.1973) (84.959, -6.6667) (86.6628, -9.7015) (88.4033, -13.6288) (90.0079, -18.0705) (91.3205, -22.607) (92.2208, -26.8073) (92.6262, -30.264) (92.4961, -32.6289) (91.8354, -33.6504) (90.7004, -33.2123) (89.2051, -31.3756) (87.5013, -28.3408) (85.7608, -24.4135) (84.1562, -19.9718) (82.8435, -15.4352) (81.9433, -11.2349) (81.5378, -7.7783) (81.642, -5.8864) (81.9588, -5.0719) (82.2686, -4.8132) (82.4468, -4.7553) knots 0 0 0 0 0 0 0.05 0.1 0.15 0.2 0.25 0.3 0.35 0.4 0.45 0.5 0.55 0.6 0.65 0.7 0.75 0.8 0.85 0.9 0.95 1 1 1 1 1 1
  line L273 (81.7693, -4.9754) -> (83.1242, -4.5352)
  line L274 (94.4427, -41.675) -> (45.4508, -25.7565)
  spline S116 degree 5 poles (100.9017, -6.4984) (100.8916, -6.5417) (100.921, -6.6469) (101.1144, -6.8586) (101.661, -7.2342) (102.753, -7.8023) (104.146, -8.4014) (105.7077, -8.9632) (107.2913, -9.4283) (108.7461, -9.7572) (109.9292, -9.9285) (110.7192, -9.9359) (111.0298, -9.7856) (110.8233, -9.4946) (110.127, -9.0882) (109.0182, -8.5994) (107.6108, -8.0666) (106.0426, -7.5331) (104.4632, -7.0456) (103.0216, -6.6533) (101.8554, -6.4023) (101.2348, -6.3432) (100.9817, -6.3871) (100.9118, -6.4551) (100.9017, -6.4984) knots 0 0 0 0 0 0 0.05 0.1 0.15 0.2 0.25 0.3 0.35 0.4 0.45 0.5 0.55 0.6 0.65 0.7 0.75 0.8 0.85 0.9 0.95 1 1 1 1 1 1
  line L275 (100.9408, -6.3312) -> (100.8626, -6.6656)
  line L276 (68.4058, -16.8961) -> (68.6762, -17.1299)
  line L277 (96.3525, -47.5528) -> (40.4508, -29.3893)
  line L278 (93.1093, -17.1055) -> (93.4154, -16.9205)
  line L279 (81.0606, -21.0158) -> (80.7428, -21.0427)
  spline S117 degree 5 poles (77.082, -11.7557) (77.1659, -11.7792) (77.3026, -11.9171) (77.4112, -12.396) (77.356, -13.5492) (76.9739, -15.6851) (76.3269, -18.2884) (75.4838, -21.0967) (74.5265, -23.8379) (73.5431, -26.2576) (72.6219, -28.1331) (71.8455, -29.2878) (71.2848, -29.6065) (70.993, -29.0523) (70.9986, -27.6843) (71.306, -25.6382) (71.8946, -23.1077) (72.7185, -20.3273) (73.704, -17.5567) (74.7503, -15.0636) (75.7456, -13.0984) (76.4132, -12.1165) (76.7997, -11.7763) (76.9982, -11.7322) (77.082, -11.7557) knots 0 0 0 0 0 0 0.05 0.1 0.15 0.2 0.25 0.3 0.35 0.4 0.45 0.5 0.55 0.6 0.65 0.7 0.75 0.8 0.85 0.9 0.95 1 1 1 1 1 1
  line L280 (76.7658, -11.6671) -> (77.3983, -11.8443)
  spline S118 degree 5 poles (76.8566, -2.9389) (76.9667, -3.0905) (77.0653, -3.4819) (76.8429, -4.327) (75.8151, -5.9189) (73.4553, -8.477) (70.2581, -11.346) (66.5296, -14.2446) (62.6207, -16.8949) (58.9042, -19.049) (55.742, -20.5028) (53.4527, -21.1098) (52.277, -20.7971) (52.3429, -19.5823) (53.6276, -17.5926) (55.9874, -15.0344) (59.1846, -12.1654) (62.9131, -9.2668) (66.822, -6.6166) (70.5385, -4.4624) (73.7007, -3.0086) (75.5322, -2.523) (76.4047, -2.5727) (76.7465, -2.7874) (76.8566, -2.9389) knots 0 0 0 0 0 0 0.05 0.1 0.15 0.2 0.25 0.3 0.35 0.4 0.45 0.5 0.55 0.6 0.65 0.7 0.75 0.8 0.85 0.9 0.95 1 1 1 1 1 1
  line L281 (76.4147, -2.3307) -> (77.2985, -3.5472)
  line L282 (76.7658, -11.6671) -> (77.3983, -11.8443)
  line L283 (90.7116, -7.5511) -> (91.0918, -6.9798)
  line L284 (45.4508, -25.7565) -> (45.4508, 25.7565)
  spline S119 degree 5 poles (93.2624, -17.013) (93.3004, -16.99) (93.4096, -16.9855) (93.6707, -17.104) (94.1968, -17.5078) (95.0746, -18.3708) (96.0748, -19.5105) (97.0917, -20.8221) (98.0234, -22.1845) (98.7857, -23.4664) (99.3143, -24.5387) (99.5654, -25.2878) (99.5185, -25.6296) (99.1778, -25.5232) (98.5762, -24.9865) (97.7687, -24.083) (96.827, -22.9091) (95.8351, -21.5826) (94.8833, -20.2311) (94.0648, -18.9813) (93.4657, -17.9497) (93.2177, -17.3778) (93.1813, -17.1234) (93.2243, -17.036) (93.2624, -17.013) knots 0 0 0 0 0 0 0.05 0.1 0.15 0.2 0.25 0.3 0.35 0.4 0.45 0.5 0.55 0.6 0.65 0.7 0.75 0.8 0.85 0.9 0.95 1 1 1 1 1 1
  line L285 (93.1093, -17.1055) -> (93.4154, -16.9205)
  line L286 (100.9408, -6.3312) -> (100.8626, -6.6656)
  point P0 (-35, 0)
  point P1 (-20, -3)
  point P2 (-9.0335, -18.0941)
  point P3 (-10.8156, -33.287)
  point P4 (-3.3272, -19.9482)
  point P5 (14.417, -14.1828)
  point P6 (28.3156, -20.5725)
  point P7 (17.9437, -9.3287)
  point P8 (17.9437, 9.3287)
  point P9 (28.3156, 20.5725)
  point P10 (14.417, 14.1828)
  point P11 (-3.3272, 19.9482)
  point P12 (-10.8156, 33.287)
  point P13 (-9.0335, 18.0941)
  point P14 (-17, 14)
  point P15 (-19, 12)
  point P16 (-18.5681, -11.8417)
  point P17 (-25, -18.1636)
  point P18 (-17.284, -14.3619)
  point P19 (5.5243, -21.3186)
  point P20 (9.5492, -29.3893)
  point P21 (8.3179, -20.8761)
  point P22 (21.9823, -1.3339)
  point P23 (30.9017, 0)
  point P24 (22.4247, 1.4597)
  point P25 (8.0615, 20.4942)
  point P26 (9.5492, 29.3893)
  point P27 (5.5414, 21.7783)
  point P28 (-25, 9)
  point P29 (-25, 7.5)
  point P30 (-16.2849, 20.9953)
  point P31 (-18.541, 25.5195)
  point P32 (-14.8583, 21.4588)
  point P33 (-16.2849, -20.9953)
  point P34 (-18.541, -25.5195)
  point P35 (-14.8583, -21.4588)
  point P36 (-25, -9)
  point P37 (-30, -9.7476)
  point P38 (-25, -7.5)
  point P39 (14.9354, -21.9758)
  point P40 (18.541, -25.5195)
  point P41 (15.817, -20.7623)
  point P42 (0.8341, -26.5576)
  point P43 (0, -31.5439)
  point P44 (-0.5925, -26.094)
  point P45 (25.5155, 7.4135)
  point P46 (30, 9.7476)
  point P47 (24.6338, 8.627)
  point P48 (25.5155, -7.4135)
  point P49 (30, -9.7476)
  point P50 (24.6338, -8.627)
  point P51 (0.8341, 26.5576)
  point P52 (0, 31.5439)
  point P53 (-0.5925, 26.094)
  point P54 (14.9354, 21.9758)
  point P55 (18.541, 25.5195)
  point P56 (15.817, 20.7623)
  point P57 (39.8583, -55.4833)
  point P58 (55, -67.1945)
  point P59 (34.0335, -58.848)
  point P60 (41.2849, -55.9468)
  point P61 (50, -84.4421)
  point P62 (50, -67.9421)
  point P63 (15.4508, -47.5528)
  point P64 (16.9385, -56.4479)
  point P65 (24.1659, -50.3845)
  point P66 (55, -86.6897)
  point P67 (19.4586, -55.1638)
  point P68 (44, -64.9421)
  point P69 (45, -73.9421)
  point P70 (-5.9017, -76.9421)
  point P71 (50, -95.1057)
  point P72 (28.3272, -56.9939)
  point P73 (24.1659, -103.4997)
  point P74 (50, -69.4421)
  point P75 (43.5681, -88.7838)
  point P76 (7.0563, -86.2707)
  point P77 (45, -79.9421)
  point P78 (60, -76.9421)
  point P79 (50, -58.7785)
  point P80 (43.541, -102.4616)
  point P81 (42.284, -91.304)
  point P82 (-3.3156, -97.5146)
  point P83 (35.8156, -110.2291)
  point P84 (25.5925, -50.848)
  point P85 (50, -85.9421)
  point P86 (41.2849, -97.9373)
  point P87 (43.541, -51.4226)
  point P88 (16.6821, -97.8182)
  point P89 (28.3272, -96.8903)
  point P90 (25, -76.9421)
  point P91 (10.583, -62.7593)
  point P92 (25, -76.9421)
  point P93 (7.0563, -67.6134)
  point P94 (39.8583, -98.4009)
  point P95 (2.5753, -75.4824)
  point P96 (10.0646, -54.9663)
  point P97 (-3.3156, -56.3696)
  point P98 (3.0177, -78.276)
  point P99 (19.4757, -98.2607)
  point P100 (42, -62.9421)
  point P101 (9.183, -56.1798)
  point P102 (0.3662, -68.3151)
  point P103 (-0.5155, -69.5286)
  point P104 (-5, -86.6897)
  point P105 (25.5925, -103.0361)
  point P106 (9.183, -97.7043)
  point P107 (-0.5155, -84.3556)
  point P108 (10.0646, -98.9179)
  point P109 (0.3662, -85.5691)
  point P110 (34.0335, -95.0362)
  point P111 (6.459, -51.4226)
  point P112 (25, -108.486)
  point P113 (-5, -67.1945)
  point P114 (35.8156, -43.6551)
  point P115 (25, -45.3982)
  point P116 (-64.8583, -73.6469)
  point P117 (-65.4508, -79.0967)
  point P118 (-65.4508, -47.5528)
  point P119 (-48.1668, -61.9147)
  point P120 (-49.1659, -68.5481)
  point P121 (-46.9098, -73.0724)
  point P122 (-50.5925, -69.0116)
  point P123 (-40.4508, -65.7164)
  point P124 (-66.2849, -74.1104)
  point P125 (-40.4508, -55.0528)
  point P126 (-40.4508, -56.5528)
  point P127 (-35.4508, -57.3004)
  point P128 (-83.3945, -56.8815)
  point P129 (-95.4509, -37.8052)
  point P130 (-73.5124, -27.0586)
  point P131 (-40.4508, -29.3893)
  point P132 (-48.4508, -33.5528)
  point P133 (-81.2679, -26.7906)
  point P134 (-70.9922, -25.7745)
  point P135 (-46.4508, -35.5528)
  point P136 (-80.3862, -25.577)
  point P137 (-95.4509, -57.3004)
  point P138 (-66.2849, -20.9953)
  point P139 (-83.9919, -22.0333)
  point P140 (-90.0847, -38.9258)
  point P141 (-40.4508, -38.5528)
  point P142 (-64.8583, -21.4588)
  point P143 (-90.9663, -54.9663)
  point P144 (-79.8678, -33.3701)
  point P145 (-79.8678, -61.7356)
  point P146 (-93.7664, -68.1253)
  point P147 (-65.4508, -47.5528)
  point P148 (-70.9751, -68.8714)
  point P149 (-54.6353, -14.2658)
  point P150 (-75, -76.9421)
  point P151 (-73.7687, -68.4289)
  point P152 (-87.8756, -46.0931)
  point P153 (-81.2679, -68.3151)
  point P154 (-96.3526, -47.5528)
  point P155 (-83.3945, -38.2242)
  point P156 (-46.9098, -22.0333)
  point P157 (-87.4331, -48.8867)
  point P158 (-45.4508, -44.5528)
  point P159 (-40.4508, -40.0528)
  point P160 (-30.4508, -47.5528)
  point P161 (-90.0847, -56.1798)
  point P162 (-93.7664, -26.9803)
  point P163 (-90.9663, -40.1393)
  point P164 (-35.4508, -37.8052)
  point P165 (-50.5925, -26.094)
  point P166 (-56.4173, -29.4587)
  point P167 (-80.3862, -69.5286)
  point P168 (-83.9919, -73.0724)
  point P169 (-49.1659, -26.5576)
  point P170 (-46.8828, -59.3945)
  point P171 (-45.4508, -50.5528)
  point P172 (-54.6353, -80.8398)
  point P173 (-62.1237, -67.501)
  point P174 (-56.4173, -65.6469)
  point P175 (-46.4508, 59.5528)
  point P176 (-75, 76.9421)
  point P177 (-73.5124, 68.047)
  point P178 (-56.4173, 65.6469)
  point P179 (-45.4508, 50.5528)
  point P180 (-70.9922, 69.3311)
  point P181 (-48.4508, 61.5528)
  point P182 (-40.4508, 65.7164)
  point P183 (-81.2679, 68.3151)
  point P184 (-65.4508, 47.5528)
  point P185 (-62.1237, 67.501)
  point P186 (-54.6353, 80.8398)
  point P187 (-90.9663, 54.9663)
  point P188 (-95.4509, 57.3004)
  point P189 (-90.0847, 56.1798)
  point P190 (-83.3945, 56.8815)
  point P191 (-90.9663, 40.1393)
  point P192 (-87.4331, 46.2189)
  point P193 (-83.3945, 38.2242)
  point P194 (-96.3526, 47.5528)
  point P195 (-87.8756, 49.0125)
  point P196 (-90.0847, 38.9258)
  point P197 (-79.8678, 61.7356)
  point P198 (-95.4509, 37.8052)
  point P199 (-80.3862, 69.5286)
  point P200 (-83.9919, 73.0724)
  point P201 (-93.7664, 68.1253)
  point P202 (-65.4508, 47.5528)
  point P203 (-65.4508, 79.0967)
  point P204 (-40.4508, 56.5528)
  point P205 (-49.1659, 68.5481)
  point P206 (-50.5925, 69.0116)
  point P207 (-66.2849, 74.1104)
  point P208 (-64.8583, 73.6469)
  point P209 (-35.4508, 57.3004)
  point P210 (-46.9098, 73.0724)
  point P211 (-40.4508, 55.0528)
  point P212 (-30.4508, 47.5528)
  point P213 (-50.5925, 26.094)
  point P214 (-65.4508, 16.009)
  point P215 (-49.1659, 26.5576)
  point P216 (-46.8828, 35.7111)
  point P217 (-70.9751, 26.2342)
  point P218 (-73.7687, 26.6767)
  point P219 (-66.2849, 20.9953)
  point P220 (-35.4508, 37.8052)
  point P221 (-64.8583, 21.4588)
  point P222 (-75, 18.1635)
  point P223 (-62.1237, 27.6046)
  point P224 (-54.6353, 14.2658)
  point P225 (-93.7664, 26.9803)
  point P226 (-80.3862, 25.577)
  point P227 (-40.4508, 38.5528)
  point P228 (-48.1668, 33.191)
  point P229 (-40.4508, 40.0528)
  point P230 (-83.9919, 22.0333)
  point P231 (-79.8678, 33.3701)
  point P232 (-45.4508, 44.5528)
  point P233 (-81.2679, 26.7906)
  point P234 (41.2849, 55.9468)
  point P235 (50, 84.4421)
  point P236 (50, 85.9421)
  point P237 (45, 73.9421)
  point P238 (34.0335, 58.848)
  point P239 (44, 88.9421)
  point P240 (42, 90.9421)
  point P241 (42.284, 62.5802)
  point P242 (43.5681, 65.1004)
  point P243 (50, 58.7785)
  point P244 (60, 76.9421)
  point P245 (9.183, 97.7043)
  point P246 (6.459, 102.4616)
  point P247 (45, 79.9421)
  point P248 (0.3662, 85.5691)
  point P249 (25.5925, 103.0361)
  point P250 (-0.5155, 84.3556)
  point P251 (19.4586, 98.7204)
  point P252 (25, 76.9421)
  point P253 (24.1659, 103.4997)
  point P254 (10.0646, 98.9179)
  point P255 (9.183, 56.1798)
  point P256 (6.459, 51.4226)
  point P257 (25.5925, 50.848)
  point P258 (25, 45.3982)
  point P259 (24.1659, 50.3845)
  point P260 (19.4757, 55.6235)
  point P261 (35.8156, 110.2291)
  point P262 (15.4508, 106.3314)
  point P263 (25, 108.486)
  point P264 (10.583, 91.1248)
  point P265 (16.9385, 97.4363)
  point P266 (35.8156, 43.6551)
  point P267 (2.5753, 78.4018)
  point P268 (16.6821, 56.066)
  point P269 (0.3662, 68.3151)
  point P270 (55, 86.6897)
  point P271 (50, 95.1057)
  point P272 (39.8583, 98.4009)
  point P273 (25, 76.9421)
  point P274 (34.0335, 95.0362)
  point P275 (28.3272, 96.8903)
  point P276 (43.541, 102.4616)
  point P277 (-3.3156, 97.5146)
  point P278 (41.2849, 97.9373)
  point P279 (28.3272, 56.9939)
  point P280 (-3.3156, 56.3696)
  point P281 (10.583, 62.7593)
  point P282 (7.0563, 67.6134)
  point P283 (3.0177, 75.6082)